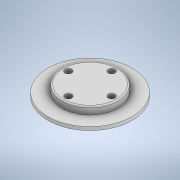
# Autodesk Inventor part: Trabajo Dibujo pieza1
Saved by Autodesk Inventor 2020 (Build 240168000, 168)
## iProperties
Created: 2021-01-05
Part Number: Trabajo Dibujo pieza1
Material: Genérico
Document SubType Name: Modeling
Designer: equipo-pcfactory
Density: 1 g/cm^3
Appearance: Valor por defecto
Author: equipo-pcfactory
Autodesk Inventor part; units mm, degrees
ref_plane "YZ Plane" through (0, 0, 0) normal (1, 0, 0) x (0, 1, 0)
ref_plane "XZ Plane" through (0, 0, 0) normal (0, 1, 0) x (-1, 0, 0)
ref_plane "XY Plane" through (0, 0, 0) normal (0, 0, 1) x (1, 0, 0)
sketch "Boceto1" plane through (0, 0, 0) normal (0, 1, 0) x (-1, 0, 0)
  circle A0 centre (0, 0) radius 62
  dimension "d0" = 124
  constraints: 1 centre point, 1 coincident
  measures "d0" diameter of A0
extrude "Extrusión1" add sketch "Boceto1" along normal blind 5
sketch "Boceto2" plane through (0, 5, 0) normal (0, 1, 0) x (1, 0, 0)
  circle A0 centre (0, 0) radius 41
  dimension "d3" = 82
  constraints: 1 centre point, 1 coincident
  measures "d3" diameter of A0
extrude "Extrusión2" add sketch "Boceto2" along normal blind 11
sketch "Boceto3" plane through (0, 16, 0) normal (0, 1, 0) x (1, 0, 0)
  circle A0 centre (-32, 0) radius 5
  circle A1 centre (0, -32) radius 5
  circle A2 centre (32, 0) radius 5
  circle A3 centre (0, 32) radius 5
  point P0 (0, 0)
  dimension "d7" = 10
  dimension "d10" = 360
  constraints: 4 centre point, 9 other
  measures "d7" diameter of A0
extrude "Extrusión3" cut sketch "Boceto3" against normal blind 4
sketch "Boceto4" plane through (32, 12, 0) normal (0, 1, 0) x (1, 0, 0)
  circle A0 centre (0, 0) radius 3.3
  circle A1 centre (-32, 32) radius 3.3
  circle A2 centre (-64, 0) radius 3.3
  circle A3 centre (-32, -32) radius 3.3
  point P0 (-32, 0)
  dimension "d14" = 6.6
  dimension "d17" = 360
  constraints: 4 centre point, 9 other
  measures "d14" diameter of A0
extrude "Extrusión4" cut sketch "Boceto4" against normal blind 12
sketch "Boceto5" plane through (0, 0, 0) normal (0, -1, 0) x (1, 0, 0)
  circle A0 centre (0, 0) radius 21
  dimension "d21" = 42
  constraints: 1 centre point, 1 coincident
  measures "d21" diameter of A0
extrude "Extrusión5" cut sketch "Boceto5" against normal blind 12
fillet "Empalme1" radius 2 1 edges at (-41, 16, 0)
fillet "Empalme2" radius 1 1 edges at (-21, 12, 0)
